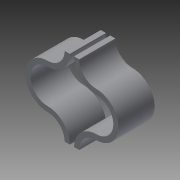
# Autodesk Inventor part: 150x0y0z_0x0y0z
Saved by Autodesk Inventor 2015 (Build 190159000, 159)
## iProperties
Created: 2016-12-15
Part Number: 150x0y0z_0x0y0z
Material: Generic
Document SubType Name: Modeling
Designer: Rudge-Top
Density: 1 g/cm^3
Appearance: Default
Author: Rudge-Top
Autodesk Inventor part; units mm, degrees
ref_plane "YZ Plane" through (0, 0, 0) normal (1, 0, 0) x (0, 1, 0)
ref_plane "XZ Plane" through (0, 0, 0) normal (0, 1, 0) x (-1, 0, 0)
ref_plane "XY Plane" through (0, 0, 0) normal (0, 0, 1) x (1, 0, 0)
sketch "Sketch1" plane through (0, 0, 0) normal (0, 1, 0) x (-1, 0, 0)
  line L0 (0, 0) -> (47.1, 0)
  line L1 (47.1, -76) -> (0, -76)
  line L2 (47.1, 0) -> (100.8601, 0) construction
  arc A0 (47.1, -59.5) -> (47.1, -16.5) centre (47.1, -38) ccw
  arc A1 (47.1, -54.5) -> (47.1, -21.5) centre (47.1, -38) ccw
  arc A2 (25.6, 0) -> (47.1, -21.5) centre (47.1, 0) ccw
  arc A3 (30.6, 0) -> (47.1, -16.5) centre (47.1, 0) ccw
  arc A4 (47.1, -54.5) -> (25.6, -76) centre (47.1, -76) ccw
  arc A5 (47.1, -59.5) -> (30.6, -76) centre (47.1, -76) ccw
  arc A6 (0, -16.5) -> (0, -59.5) centre (0, -38) ccw
  arc A7 (0, -21.5) -> (0, -54.5) centre (0, -38) ccw
  arc A8 (0, -21.5) -> (21.5, 0) centre (0, 0) ccw
  arc A9 (0, -16.5) -> (16.5, 0) centre (0, 0) ccw
  arc A10 (21.5, -76) -> (0, -54.5) centre (0, -76) ccw
  arc A11 (16.5, -76) -> (0, -59.5) centre (0, -76) ccw
  dimension "d0" = 47.1
  dimension "d1" = 76
  dimension "d5" = 43
  dimension "d6" = 33
  dimension "d8" = 43
  constraints: 24 point on circle, 12 centre point, 8 point on line, 6 coincident, 6 end point, 2 horizontal, 1 parallel
  measures "d0" distance of L1.start L1.end
  measures "d1" distance of L0.end L1.start
  measures "d5" diameter of A0
  measures "d6" diameter of A1
  measures "d8" diameter of A2
extrude "Extrusion1" add sketch "Sketch1" along normal blind 35 contours L0 A8 A7 A10 L1 A11 A6 A9 | L0 A3 A0 A5 L1 A4 A1 A2
body "Solid1"
